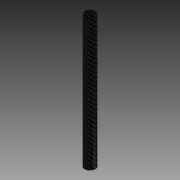
# Autodesk Inventor part: ROD001 - Rod 20x18mm
Saved by Autodesk Inventor 2015 SP1 (Build 190203100, 203)
## iProperties
Created: 2015-05-12
Part Number: ROD001 - Rod 20x18mm
Material: Generic
Document SubType Name: Modeling
Designer: rhornbak
Density: 1 g/cm^3
Appearance: Default
Author: rhornbak
Autodesk Inventor part; units mm, degrees
ref_plane "YZ Plane" through (0, 0, 0) normal (1, 0, 0) x (0, 1, 0)
ref_plane "XZ Plane" through (0, 0, 0) normal (0, 1, 0) x (-1, 0, 0)
ref_plane "XY Plane" through (0, 0, 0) normal (0, 0, 1) x (1, 0, 0)
sketch "Sketch1" plane through (0, 0, 0) normal (0, 0, 1) x (1, 0, 0)
  circle A0 centre (0, 0) radius 8.95
  circle A1 centre (0, 0) radius 10.025
  dimension "RodInner" = 17.9
  dimension "RodDia" = 20.05
  constraints: 2 centre point, 2 coincident
  measures "RodInner" diameter of A0
  measures "RodDia" diameter of A1
extrude "Extrusion1" add sketch "Sketch1" along normal mid plane 250
body "Solid1"
